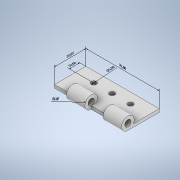
# Autodesk Inventor part: Dobradiça
Saved by Autodesk Inventor 2021 (Build 250183000, 183)
## iProperties
Created: 2021-08-09
Part Number: Dobradiça
Material: Generic
Document SubType Name: Modeling
Designer: guilh
Density: 1 g/cm^3
Appearance: Default
Author: guilh
Autodesk Inventor part; units mm, degrees
ref_plane "YZ Plane" through (0, 0, 0) normal (1, 0, 0) x (0, 1, 0)
ref_plane "XZ Plane" through (0, 0, 0) normal (0, 1, 0) x (-1, 0, 0)
ref_plane "XY Plane" through (0, 0, 0) normal (0, 0, 1) x (1, 0, 0)
sketch "Sketch1" plane through (0, 0, 0) normal (0, 1, 0) x (-1, 0, 0)
  line L0 (0, 0) -> (0, -30)
  line L1 (0, -30) -> (70, -30)
  line L2 (70, -30) -> (70, 0)
  line L3 (70, 0) -> (0, 0)
  line L4 (70, -30) -> (70, -20)
  line L5 (70, -20) -> (52.5, -20)
  line L6 (52.5, -20) -> (35, -20)
  line L7 (35, -20) -> (17.5, -20)
  circle A0 centre (52.5, -20) radius 2.5
  circle A1 centre (35, -20) radius 2.5
  circle A2 centre (17.5, -20) radius 2.5
  dimension "d0" = 30
  dimension "d1" = 70
  dimension "d2" = 10
  dimension "d3" = 17.5
  dimension "d4" = 17.5
  dimension "d5" = 17.5
  dimension "d6" = 5
  dimension "d7" = 5
  dimension "d8" = 5
  constraints: 16 end point, 4 perpendicular, 3 centre point, 3 coincident, 3 point on line, 1 vertical
  measures "d0" distance of L0.start L0.end
  measures "d1" distance of L0.end L1.end
  measures "d2" distance of L1.end L4.end
  measures "d3" distance of L4.end L5.end
  measures "d4" distance of L5.end L6.end
  measures "d5" distance of L6.end L7.end
  measures "d6" diameter of A0
  measures "d7" diameter of A1
  measures "d8" diameter of A2
extrude "Extrusion1" add sketch "Sketch1" along normal blind 3
sketch "Sketch2" plane through (0, 0, 0) normal (1, 0, 0) x (0, 0, -1)
  line L0 (0, 3) -> (30, 3) projected
  circle A0 centre (0, 6) radius 3
  line L1 (0, 0) -> (0, 3) projected
  circle A1 centre (0, 6) radius 6
  constraints: 1 centre point, 1 coincident, 1 vertical alignment, 2 other
extrude "Extrusion2" add sketch "Sketch2" against normal blind 70 contours L1 A1 L0 | A0 | L0 A1 L1
sketch "Sketch3" plane through (0, 0, -30) normal (1, 0, 0) x (0, 0, -1)
  line L0 (-30, 0) -> (0, 0) projected
  line L1 (-30, 0) -> (-30, 6)
  circle A0 centre (-30, 6) radius 3
  dimension "d14" = 6
  dimension "d15" = 6
  constraints: 2 end point, 1 centre point, 1 coincident, 1 vertical
  measures "d14" distance of L0.start L1.end
  measures "d15" diameter of A0
extrude "Extrusion3" cut sketch "Sketch3" against normal blind 70
sketch "Sketch4" plane through (0, 0, -30) normal (0, 0, -1) x (-1, 0, 0)
  line L0 (0, 0) -> (70, 0) projected
  line L1 (0, 0) -> (0, 3)
  line L2 (0, 3) -> (70, 3) projected
  line L3 (0, 3) -> (17.5, 3)
  line L4 (17.5, 3) -> (35, 3)
  line L5 (35, 3) -> (52.5, 3)
  line L6 (52.5, 3) -> (70, 3)
  line L7 (70, 0) -> (70, 12) projected
  line L8 (70, 3) -> (70, 12)
  line L9 (70, 12) -> (52.5, 12)
  line L10 (0, 12) -> (70, 12) projected
  line L11 (52.5, 3) -> (52.5, 12)
  line L12 (17.5, 3) -> (17.5, 12)
  line L13 (17.5, 12) -> (35, 12)
  line L14 (35, 12) -> (35, 3)
  dimension "d18" = 17.5
  dimension "d19" = 17.5
  dimension "d20" = 17.5
  constraints: 22 end point, 6 point on line, 2 collinear, 2 perpendicular, 1 midpoint, 1 parallel, 1 vertical
  measures "d18" distance of L1.end L3.end
  measures "d19" distance of L3.end L4.end
  measures "d20" distance of L4.end L5.end
extrude "Extrusion4" cut sketch "Sketch4" against normal blind 70 contours L2 L11 L9 L7 | L12 L10 L14 L2
sketch "Sketch5" plane through (0, 3, 0) normal (0, 1, 0) x (1, 0, 0)
  line L0 (-17.5, -5.1962) -> (-35, -5.1962) projected
  line L1 (-35, 6) -> (-35, -6) projected
  line L2 (-35, 0) -> (-35, -5.1962) projected
  line L3 (-35, -5.1962) -> (-17.5, -5.1962)
  line L4 (-17.5, -5.1962) -> (-17.5, 0)
  line L5 (-17.5, 0) -> (-35, 0)
  line L6 (-35, 5.1962) -> (-35, 0) projected
  line L7 (-35, 0) -> (-35, -5.1962)
  line L8 (-52.5, -5.1962) -> (-70, -5.1962) projected
  line L9 (-52.5, -5.1962) -> (-70, -5.1962)
  line L10 (-70, 0) -> (-70, -5.1962) projected
  line L11 (-70, -5.1962) -> (-70, 0)
  line L12 (-70, 0) -> (-52.5, 0)
  line L13 (-70, 0) -> (0, 0) projected
  line L14 (-52.5, 0) -> (-52.5, -5.1962) projected
  line L15 (-52.5, 5.1962) -> (-52.5, 0) projected
  line L16 (-52.5, -5.1962) -> (-52.5, 0)
  dimension "d24" = 17.5
  constraints: 16 end point, 2 horizontal, 2 perpendicular, 1 collinear, 1 midpoint, 1 point on line, 1 vertical
  measures "d24" distance of L0.end L0.start
extrude "Extrusion5" cut sketch "Sketch5" against normal blind 70
body "Solid1"
